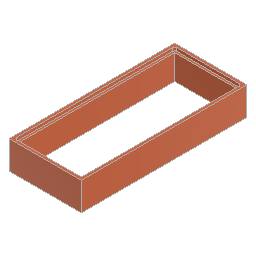
Dry-Erase-Marker-Holder (Autodesk Fusion 360 design; units mm, degrees)
Autodesk Fusion 360 part; units mm, degrees
sketch "Sketch1" plane through (0, 0, 3.175) normal (0, 0, 1) x (-1, 0, 0)
  line L0 (0, 0) -> (0, 297.942)
  line L1 (0, 297.942) -> (-407.924, 297.942)
  line L2 (-407.924, 297.942) -> (-407.924, 0)
  line L3 (-407.924, 0) -> (0, 0)
  line L4 (0, 0) -> (-65, 0)
  line L5 (-65, 0) -> (-65, 148.97)
  line L6 (-65, 148.97) -> (0, 148.97)
  line L7 (0, 148.97) -> (0, 0)
  line L8 (-4.5, 144.47) -> (-4.5, 4.5)
  line L9 (-4.5, 4.5) -> (-60.5, 4.5)
  line L10 (-60.5, 4.5) -> (-60.5, 144.47)
  line L11 (-60.5, 144.47) -> (-4.5, 144.47)
  dimension "d100" = 65
  dimension "d101" = 148.97
  dimension "d102" = 4.5
  constraint horizontal L4
  constraint vertical L5
  constraint horizontal L6
  constraint vertical L7
  constraint coincident L0.start L3.end
  measures "d100" distance of L0.start L4.end
  measures "d101" distance of L0.start L6.end
extrude "Extrude1" add sketch "Sketch1" along normal blind 25.4 contours L0 L3 L4 L5 L6 L7
sketch "Sketch2" plane through (0, 0, 28.575) normal (0, 0, 1) x (-1, 0, 0)
  line L0 (-60.5, 4.5) -> (-60.5, 144.47)
  line L1 (-60.5, 144.47) -> (-4.5, 144.47)
  line L2 (-4.5, 144.47) -> (-4.5, 4.5)
  line L3 (-4.5, 4.5) -> (-60.5, 4.5)
  line L4 (0, 148.97) -> (-65, 148.97)
  line L5 (-65, 148.97) -> (-65, 0)
  line L6 (-65, 0) -> (0, 0)
  line L7 (0, 0) -> (0, 148.97)
  line L8 (-60.5, 4.5) -> (-60.5, 144.47)
  line L9 (-60.5, 144.47) -> (-4.5, 144.47)
  line L10 (-4.5, 144.47) -> (-4.5, 4.5)
  line L11 (-4.5, 4.5) -> (-60.5, 4.5)
  line L12 (-4.5, 2.5) -> (-60.5, 2.5)
  line L13 (-62.5, 4.5) -> (-62.5, 144.47)
  line L14 (-60.5, 146.47) -> (-4.5, 146.47)
  line L15 (-2.5, 144.47) -> (-2.5, 4.5)
  arc A0 (-60.5, 146.47) -> (-62.5, 144.47) centre (-60.5, 144.47) ccw
  arc A1 (-2.5, 144.47) -> (-4.5, 146.47) centre (-4.5, 144.47) ccw
  arc A2 (-4.5, 2.5) -> (-2.5, 4.5) centre (-4.5, 4.5) ccw
  arc A3 (-62.5, 4.5) -> (-60.5, 2.5) centre (-60.5, 4.5) ccw
  dimension "d106" = 2
  constraint tangent L14 A0
  constraint tangent L13 A0
  constraint tangent L14 A1
  constraint tangent L15 A1
  constraint equal A0 A1
  constraint tangent L15 A2
  constraint tangent L12 A2
  constraint equal A0 A2
  constraint tangent L12 A3
  constraint tangent L13 A3
  constraint equal A0 A3
  measures "d106" radius of A0
extrude "Extrude2" cut sketch "Sketch2" against normal blind 3 contours L12 L13 L14 L15 A0 A1 A2 A3
equation "d101 = DigitalStorageLength"
equation "d102 = ComponentWallWidth + 0.5 mm"
equation "DigitalStorageLength = 148.97 mm"
equation "ComponentWallWidth = 4 mm"
